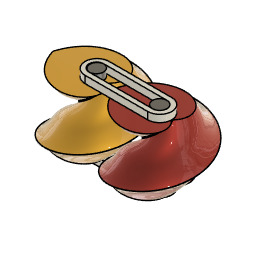
Bonus v1 (Autodesk Fusion 360 design; units mm, degrees)
Autodesk Fusion 360 part; units mm, degrees
sketch "Sketch1" plane through (0, 0, 0) normal (0, 0, 1) x (1, 0, 0)
  spline S0 degree 5 poles (0.4891, 1.5341) (2.5688, 7.9851) (7.3005, 21.1368) (15.928, 40.8354) (30.8894, 66.5381) (57.2477, 95.7536) (92.9898, 119.1223) (137.1612, 132.5945) (185.1229, 131.36) (226.2877, 110.9383) (252.263, 77.2952) (256.6274, 46.0408) (248.9853, 23.6252) (239.0525, 9.7581) (233.2226, 3.3707) knots 0.004539 0.004539 0.004539 0.004539 0.004539 0.004539 0.1 0.2 0.3 0.4 0.5 0.6 0.7 0.8 0.9 0.990396 0.990396 0.990396 0.990396 0.990396 0.990396
  line L0 (125, 130) -> (185, 130)
  line L1 (0, 0) -> (320, 0) construction
  circle A0 centre (180, 0) radius 30
  spline S1 degree 5 poles (0.4891, -1.5341) (2.5688, -7.9851) (7.3005, -21.1368) (15.928, -40.8354) (30.8894, -66.5381) (57.2477, -95.7536) (92.9898, -119.1223) (137.1612, -132.5945) (185.1229, -131.36) (226.2877, -110.9383) (252.263, -77.2952) (256.6274, -46.0408) (248.9853, -23.6252) (239.0525, -9.7581) (233.2226, -3.3707) knots 0.004539 0.004539 0.004539 0.004539 0.004539 0.004539 0.1 0.2 0.3 0.4 0.5 0.6 0.7 0.8 0.9 0.990396 0.990396 0.990396 0.990396 0.990396 0.990396
  line L2 (125, -130) -> (185, -130)
  arc A1 (0.4891, 1.5341) -> (0.4891, -1.5341) centre (5.248, 0) ccw
  arc A2 (233.2226, 3.3707) -> (233.2226, -3.3707) centre (236.9156, 0) ccw
  point P0 (155, 130)
  point P1 (230, 0)
  point P2 (155, -130)
  dimension "d1" = 230
  dimension "d2" = 130
  dimension "d3" = 75
  dimension "d4" = 60
  dimension "d9" = 60
  dimension "d10" = 50
  dimension "d11" = 5
  dimension "d12" = 5
  constraint coincident L1.start origin
  constraint midpoint P0 L0
  constraint horizontal L0
  constraint horizontal L1.start P1
  constraint horizontal L1
  constraint coincident L1 A0.centre
  constraint symmetric P0 L1 P2
  constraint symmetric L0.start L1 L2.start
  constraint symmetric L0.end L1 L2.end
  constraint tangent S0 A1
  constraint tangent S1 A1
  constraint tangent S0 A2
  constraint tangent S1 A2
  measures "d1" distance of L1.start P1
  measures "d2" vertical distance of P0 P1
  measures "d3" horizontal distance of P0 P1
  measures "d4" distance of L0.start L0.end
  measures "d9" diameter of A0
  measures "d10" distance of P1 A0.centre
  measures "d11" radius of A1
  measures "d12" radius of A2
sketch "Sketch2" plane through (0, 0, 0) normal (0, 1, 0) x (1, 0, 0)
  line L0 (180, 0) -> (180, -240)
  dimension "d13" = 240
  constraint vertical L0
  measures "d13" distance of L0.start L0.end
sweep "Sweep1" add twist angle 360 profiles "Sketch1" path "Sketch2" along L0 section 1 contours S0 S1 A1 A2 makes body 1
extrude "Extrude1" add sketch "Sketch1" along normal blind 270 and the other way blind 30 separate body contours A0 makes body 2
copy_body "CopyPasteBodies1" bodies 2 1 makes body 3 makes body 4
move_body "Move1" bodies 3 4 to x (1, 0, 0) y (0, 1, 0) z (0, 0, 1) at (-263.5, 0, 0)
sketch "Sketch3" plane through (0, 0, 240) normal (0, 0, 1) x (-1, 0, 0)
  circle A0 centre (-180, 0) radius 30
  arc A1 (-0.4891, -1.5341) -> (-0.4891, 1.5341) centre (-5.248, 0) ccw
  spline S0 degree 5 poles (-0.4891, 1.5341) (-2.5688, 7.9851) (-7.3005, 21.1368) (-15.928, 40.8354) (-30.8894, 66.5381) (-57.2477, 95.7536) (-92.9898, 119.1223) (-137.1612, 132.5945) (-185.1229, 131.36) (-226.2877, 110.9383) (-252.263, 77.2952) (-256.6274, 46.0408) (-248.9853, 23.6252) (-239.0525, 9.7581) (-233.2226, 3.3707) knots 0.004539 0.004539 0.004539 0.004539 0.004539 0.004539 0.1 0.2 0.3 0.4 0.5 0.6 0.7 0.8 0.9 0.990396 0.990396 0.990396 0.990396 0.990396 0.990396
  arc A2 (-233.2226, -3.3707) -> (-233.2226, 3.3707) centre (-236.9156, 0) ccw
  spline S1 degree 5 poles (-233.2226, -3.3707) (-239.0525, -9.7581) (-248.9853, -23.6252) (-256.6274, -46.0408) (-252.263, -77.2952) (-226.2877, -110.9383) (-185.1229, -131.36) (-137.1612, -132.5945) (-92.9898, -119.1223) (-57.2477, -95.7536) (-30.8894, -66.5381) (-15.928, -40.8354) (-7.3005, -21.1368) (-2.5688, -7.9851) (-0.4891, -1.5341) knots -0.990396 -0.990396 -0.990396 -0.990396 -0.990396 -0.990396 -0.9 -0.8 -0.7 -0.6 -0.5 -0.4 -0.3 -0.2 -0.1 -0.004539 -0.004539 -0.004539 -0.004539 -0.004539 -0.004539
  line L0 (80, 30) -> (-180, 30)
  arc A3 (-180, 30) -> (-180, -30) centre (-180, 0) ccw
  line L1 (-180, -30) -> (80, -30)
  arc A4 (80, -30) -> (80, 30) centre (80, 0) ccw
  line L2 (80, 0) -> (-180, 0) construction
  line L3 (80, 50) -> (-180, 50)
  arc A5 (-180, 50) -> (-180, -50) centre (-180, 0) ccw
  line L4 (-180, -50) -> (80, -50)
  arc A6 (80, -50) -> (80, 50) centre (80, 0) ccw
  dimension "d24" = 60
  dimension "d25" = 20
  constraint tangent L0 A3
  constraint tangent A3 L1
  constraint parallel L0 L1
  constraint tangent L1 A4
  constraint tangent L0 A4
  constraint coincident A0.centre A3.centre
  constraint horizontal L2
  measures "d24" diameter of A3
extrude "Extrude2" add sketch "Sketch3" along normal blind 30 separate body contours A0 S0 S1 L0 A3 L1 L3 A5 L4 | S0 S1 L0 L1 A4 L3 L4 A6 makes body 5
copy_body "CopyPasteBodies2" bodies 5 makes body 6
move_body "Move2" bodies 6 to x (1, 0, 0) y (0, 1, 0) z (0, 0, 1) at (0, 0, -270)
copy_body "Body->Comp1" bodies 1 removing the originals makes body 7 in component "Component"
copy_body "Body->Comp2" bodies 2 removing the originals makes body 8 in component "Component'"
copy_body "Body->Comp3" bodies 3 removing the originals makes body 9 in component "Component''"
copy_body "Body->Comp4" bodies 4 removing the originals makes body 10 in component "Component'''"
copy_body "Body->Comp5" bodies 5 removing the originals makes body 11 in component "Component''''"
copy_body "Body->Comp6" bodies 6 removing the originals makes body 12 in component "Component'''''"
component "Component" placed x (1, 0, 0) y (0, 1, 0) z (0, 0, 1) at (0, 0, 0)
component "Component'" placed x (1, 0, 0) y (0, 1, 0) z (0, 0, 1) at (0, 0, 0)
component "Component''" placed x (1, 0, 0) y (0, 1, 0) z (0, 0, 1) at (0, 0, 0)
component "Component'''" placed x (1, 0, 0) y (0, 1, 0) z (0, 0, 1) at (0, 0, 0)
component "Component''''" placed x (1, 0, 0) y (0, 1, 0) z (0, 0, 1) at (0, 0, 0)
component "Component'''''" placed x (1, 0, 0) y (0, 1, 0) z (0, 0, 1) at (0, 0, 0)
